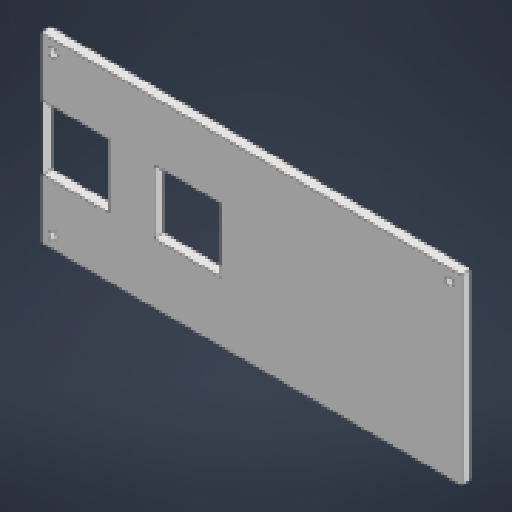
# Autodesk Inventor part: backplate_lvl202x01
Saved by Autodesk Inventor 2024 (Build 280153000, 153)
## iProperties
Created: 2026-05-08
Part Number: backplate_lvl202x01
Material: Generic
Document SubType Name: Modeling
Designer: schar
Density: 1 g/cm^3
Appearance: Default
Author: schar
Autodesk Inventor part; units mm, degrees
ref_plane "YZ Plane" through (0, 0, 0) normal (1, 0, 0) x (0, 1, 0)
ref_plane "XZ Plane" through (0, 0, 0) normal (0, 1, 0) x (-1, 0, 0)
ref_plane "XY Plane" through (0, 0, 0) normal (0, 0, 1) x (1, 0, 0)
sketch "Sketch1" plane through (0, 0, 0) normal (0, 0, 1) x (1, 0, 0)
  line L0 (-112.7024, 42.5741) -> (-128.5024, 42.5741) projected
  line L1 (-112.2524, 27.0241) -> (-112.2524, 42.1241) projected
  line L2 (-100.8524, 42.2341) -> (-100.8524, 27.1341) projected
  line L3 (-84.6024, 42.6841) -> (-100.4024, 42.6841) projected
  line L4 (-84.1524, 27.1341) -> (-84.1524, 32.1691) projected
  line L5 (-100.4024, 26.6841) -> (-84.6024, 26.6841) projected
  line L6 (-128.5024, 26.5741) -> (-112.7024, 26.5741) projected
  line L7 (-128.9524, 32.0591) -> (-128.9524, 27.0241) projected
  circle A0 centre (-126.4024, 54.4141) radius 1.1 projected
  circle A1 centre (-126.4024, 14.4141) radius 1.1 projected
  line L8 (-129.6024, 11.2141) -> (-129.6024, 57.6141) projected
  line L9 (-23.2024, 11.2141) -> (-129.6024, 11.2141) projected
  line L10 (-23.2024, 57.6141) -> (-23.2024, 11.2141) projected
  line L11 (-129.6024, 57.6141) -> (-23.2024, 57.6141) projected
  line L12 (-112.7024, 26.5741) -> (-108.9398, 26.5741)
  line L13 (-112.2524, 27.0241) -> (-112.2524, 26.5741)
  line L14 (-128.5024, 42.5741) -> (-131.0464, 42.5741)
  line L15 (-128.9524, 32.0591) -> (-128.9524, 42.5741)
  line L16 (-128.9524, 42.5741) -> (-112.2524, 42.5741)
  line L17 (-112.2524, 42.5741) -> (-112.2524, 26.5741)
  line L18 (-112.2524, 26.5741) -> (-128.9524, 26.5741)
  line L19 (-128.9524, 26.5741) -> (-128.9524, 42.5741)
  line L20 (-100.4024, 26.6841) -> (-102.0076, 26.6841)
  line L21 (-100.8524, 27.1341) -> (-100.8524, 26.6841)
  line L22 (-84.1524, 32.1691) -> (-84.1524, 43.4133)
  line L23 (-84.6024, 42.6841) -> (-84.1524, 42.6841)
  line L24 (-84.1524, 42.6841) -> (-100.8524, 42.6841)
  line L25 (-100.8524, 42.6841) -> (-100.8524, 26.6841)
  line L26 (-100.8524, 26.6841) -> (-84.1524, 26.6841)
  line L27 (-84.1524, 26.6841) -> (-84.1524, 42.6841)
  line L28 (-23.2024, 57.6141) -> (-26.4024, 57.6141)
  line L29 (-26.4024, 57.6141) -> (-26.4024, 54.4141)
  circle A2 centre (-26.4024, 54.4141) radius 1.1
  line L30 (-23.2024, 11.2141) -> (-21.0735, 11.2141)
  line L31 (-21.0735, 11.2141) -> (-21.0735, 8.0141)
  circle A3 centre (-21.0735, 8.0141) radius 1.1
  line L32 (-23.4024, 57.4141) -> (-23.4024, 11.4141)
  line L33 (-23.4024, 11.4141) -> (-129.4024, 11.4141)
  line L34 (-129.4024, 11.4141) -> (-129.4024, 57.4141)
  line L35 (-129.4024, 57.4141) -> (-23.4024, 57.4141)
  point P0 (0, 0)
  point P1 (-128.9524, 32.0583)
  point P2 (-46.5566, -2.8057)
  point P3 (-1.7566, -2.6957)
  dimension "d0" = 3.2
  dimension "d1" = 3.2
  dimension "d2" = 2.2
  dimension "d3" = 3.2
  dimension "d4" = 2.2
  dimension "d7" = 0.2
  constraints: 48 end point, 6 perpendicular, 6 point on line, 4 horizontal, 4 parallel, 3 collinear, 3 vertical, 2 centre point, 2 coincident, 3 other
  measures "d0" distance of L10.start L28.end
  measures "d1" distance of L28.end L29.end
  measures "d2" diameter of A2
  measures "d3" distance of L30.end L31.end
  measures "d4" diameter of A3
  measures "d7" distance between parallel lines of L11 L35
extrude "Extrusion1" add sketch "Sketch1" against normal blind 2.5 contours L34 L35 L32 L33
sketch "Sketch2" plane through (0, 0, 0) normal (0, 0, 1) x (1, 0, 0)
  circle A0 centre (-26.4024, 14.4141) radius 1.1 projected
  point P0 (0, 0)
extrude "Extrusion2" cut sketch "Sketch2" against normal blind 2.5
body "Solid1"
